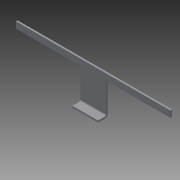
# Autodesk Inventor part: Pneumatic Puller Mount
Saved by Autodesk Inventor 2013 (Build 170138000, 138)
## iProperties
Created: 2013-02-01
Part Number: Pneumatic Puller Mount
Material: Generic
Document SubType Name: Sheet Metal
Designer: actoennies
Density: 1 g/cm^3
Sheet Metal Rule: Default
Author: actoennies
Autodesk Inventor part; units mm, degrees
ref_plane "YZ Plane" through (0, 0, 0) normal (1, 0, 0) x (0, 1, 0)
ref_plane "XZ Plane" through (0, 0, 0) normal (0, 1, 0) x (-1, 0, 0)
ref_plane "XY Plane" through (0, 0, 0) normal (0, 0, 1) x (1, 0, 0)
sketch "Sketch1" plane through (0, 0, 0) normal (0, 1, 0) x (-1, 0, 0)
  line L0 (0, 0) -> (0, 12.7)
  line L1 (0, 12.7) -> (50.8, 12.7)
  line L2 (50.8, 12.7) -> (50.8, 0)
  line L3 (50.8, 0) -> (0, 0)
  dimension "d0" = 12.7
  dimension "d1" = 50.8
  measures "d0" distance of L0.start L0.end
  measures "d1" distance of L0.end L1.end
sketch "Sketch3" plane through (-50.8, 76.2, -3.175) normal (0, 0, 1) x (1, 0, 0)
  line L0 (50.8, 0) -> (50.8, -69.85)
  line L1 (0, 0) -> (0, -69.85)
  line L2 (50.8, 0) -> (177.8, 0)
  line L3 (177.8, 0) -> (177.8, -12.7)
  line L4 (177.8, -12.7) -> (50.8, -12.7)
  line L5 (0, 0) -> (-127, 0)
  line L6 (-127, 0) -> (-127, -12.7)
  line L7 (-127, -12.7) -> (0, -12.7)
  point P0 (50.8, -76.2)
  dimension "d13" = 127
  dimension "d14" = 12.7
  dimension "d15" = 127
  measures "d13" distance of L0.start L2.end
  measures "d14" distance of L2.end L3.end
  measures "d15" distance of L1.start L5.end
extrude "Plate1" add sketch "Sketch1" along normal blind 3.175
sketch "Sketch2" plane through (-50.8, 6.35, -3.175) normal (0, 0, -1) x (-1, 0, 0)
  line L0 (-50.8, 0) -> (0, 0)
  line L1 (0, 0) -> (0, 69.85)
  line L2 (0, 69.85) -> (-50.8, 69.85)
  line L3 (-50.8, 69.85) -> (-50.8, 0)
  constraints: 6 end point, 1 horizontal, 1 perpendicular, 1 vertical
edge flange "Flange1" height 76.2 angle 90 thickness 3.175 bend radius 3.175 thickness toward (0, 0, -1) relief straight relief width 3.175 relief depth 1.5875 edges at (-25.4, 3.175, 0) wall of the first edge with corners at (0, 6.35, -3.175) (-50.8, 6.35, -3.175) (-50.8, 76.2, -3.175) (0, 76.2, -3.175)
bend "Bend1"
corner "Corner1"
sheet face with bend "Face2" sketch "Sketch3" thickness 3.175 toward (0, 0, -1) bend radius 3.175 relief straight relief width 3.175 relief depth 1.5875
bend "Bend2"
equation "\"d3\" = BendReliefWidth"
equation "\"d4\" = BendReliefDepth"
equation "\"d5\" = MinimumRemnant"
equation "\"d6\" = BendRadius"
equation "\"d9\" = BendRadius"
equation "\"d10\" = CornerReliefSize"
equation "\"d11\" = GapSize"
equation "\"d12\" = JacobiRadiusSize"
equation "\"d16\" = BendRadius"
equation "\"d17\" = BendReliefWidth"
equation "\"d19\" = MinimumRemnant"
equation "\"d18\" = BendReliefDepth"
equation "\"d20\" = BendRadius"
equation "\"BendRadius\" = Thickness"
equation "\"BendReliefWidth\" = Thickness"
equation "\"BendReliefDepth\" = 0.5 * Thickness"
equation "\"CornerReliefSize\" = 4 * Thickness"
equation "\"MinimumRemnant\" = 2 * Thickness"
equation "\"TransitionRadius\" = BendRadius"
equation "\"JacobiRadiusSize\" = BendRadius"
equation "\"GapSize\" = Thickness"
equation "\"d2\" = BendRadius"
equation "\"Thickness\" = 3.175"
body "Solid1"
